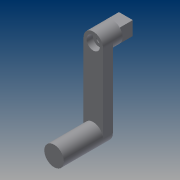
# Autodesk Inventor part: Crank
Saved by Autodesk Inventor 2016 (Build 200138000, 138)
## iProperties
Created: 2015-04-28
Part Number: Crank
Material: ABS Plastic
Document SubType Name: Modeling
Designer: Trevor
Density: 1.06 g/cm^3
Appearance: Smooth - White
d_key: 0.250 in
l_key: 0.265 in
t: 0.188 in
Author: Trevor
Autodesk Inventor part; units mm, degrees
ref_plane "YZ Plane" through (0, 0, 0) normal (1, 0, 0) x (0, 1, 0)
ref_plane "XZ Plane" through (0, 0, 0) normal (0, 1, 0) x (-1, 0, 0)
ref_plane "XY Plane" through (0, 0, 0) normal (0, 0, 1) x (1, 0, 0)
sketch "Sketch1" plane through (0, 0, 0) normal (0, 0, 1) x (1, 0, 0)
  line L0 (-3.3676, 3.3676) -> (3.3676, 3.3676)
  line L1 (3.3676, 3.3676) -> (3.3676, -3.3676)
  line L2 (3.3676, -3.3676) -> (-3.3676, -3.3676)
  line L3 (-3.3676, -3.3676) -> (-3.3676, 3.3676)
  line L4 (-3.3676, 3.3676) -> (3.3676, -3.3676) construction
  line L5 (3.3676, 3.3676) -> (-3.3676, -3.3676) construction
  point P0 (0, 0)
  dimension "d0" = 6.7352
  constraints: 12 end point, 2 midpoint, 2 parallel, 2 perpendicular, 1 horizontal
  measures "d0" distance of L0.end L1.end
extrude "Extrusion1" add sketch "Sketch1" along normal blind 6.35
sketch "Sketch2" plane through (0, 0, 6.35) normal (0, 0, 1) x (1, 0, 0)
  line L0 (3.3676, -3.3676) -> (3.3676, 3.3676) projected
  line L1 (-3.3676, -3.3676) -> (3.3676, -3.3676) projected
  line L2 (3.3676, 3.3676) -> (-3.3676, 3.3676) projected
  line L3 (-3.3676, 3.3676) -> (-3.3676, -3.3676) projected
  circle A0 centre (0, 0) radius 4.7625
  constraints: 1 coincident, 3 other
extrude "Extrusion2" add sketch "Sketch2" along normal blind 4.7625
sketch "Sketch3" plane through (0, 0, 11.1125) normal (0, 0, 1) x (1, 0, 0)
  circle A0 centre (0, 0) radius 4.7625 projected
  line L0 (0, 0) -> (0, -38.1) construction
  line L1 (-4.7625, 0) -> (-4.7625, -38.1)
  line L2 (4.7625, -38.1) -> (4.7625, 0)
  arc A1 (4.7625, 0) -> (-4.7625, 0) centre (0, 0) ccw
  arc A2 (-4.7625, -38.1) -> (4.7625, -38.1) centre (0, -38.1) ccw
  circle A3 centre (0, 0) radius 4.7625 projected
  point P0 (0, -19.05)
  dimension "d5" = 38.1
  constraints: 8 end point, 4 point on circle, 4 tangent, 2 centre point, 1 horizontal alignment, 1 midpoint, 1 parallel, 1 vertical, 1 other
  measures "d5" distance of L0.start L0.end
extrude "Extrusion3" add sketch "Sketch3" along normal blind 4.7625
sketch "Sketch4" plane through (0, 0, 15.875) normal (0, 0, 1) x (1, 0, 0)
  circle A0 centre (0, -38.1) radius 4.7625
  line L0 (4.7625, 0) -> (4.7625, -38.1) projected
  arc A1 (-4.7625, -38.1) -> (4.7625, -38.1) centre (0, -38.1) ccw projected
  line L1 (-4.7625, -38.1) -> (-4.7625, 0) projected
  arc A2 (4.7625, 0) -> (-4.7625, 0) centre (0, 0) ccw projected
  arc A3 (-4.7625, -38.1) -> (4.7625, -38.1) centre (0, -38.1) ccw projected
  constraints: 1 horizontal alignment, 3 other
extrude "Extrusion4" add sketch "Sketch4" along normal blind 19.05 contours A0
sketch "Sketch5" plane through (-3.3676, -3.3676, 0) normal (-1, 0, 0) x (0, 0, 1)
  point P0 (0, 3.3676)
sketch "Sketch6" plane through (0, 0, 15.875) normal (0, 0, 1) x (1, 0, 0)
  circle A0 centre (0, 0) radius 4.7625
  line L0 (4.7625, 0) -> (4.7625, -38.1) projected
  arc A1 (-4.7625, -38.1) -> (4.7625, -38.1) centre (0, -38.1) ccw projected
  arc A2 (4.7625, -38.1) -> (-4.7625, -38.1) centre (0, -38.1) ccw projected
  arc A3 (4.7625, 0) -> (-4.7625, 0) centre (0, 0) ccw projected
  line L1 (-4.7625, -38.1) -> (-4.7625, 0) projected
  constraints: 2 coincident, 1 horizontal alignment, 2 other
hole "Hole1" at (0, 0, 15.875) direction (0, 0, -1) diameter 3.4036 end through all counterbore diameter 6.5024 counterbore depth 2.9972 clearance for "Socket Head Cap Screw" size "M3" standard "Ansi Metric M Profile"
equation "\"d0\" = l_key"
equation "\"d1\" = d_key"
equation "\"d6\" = t"
equation "\"d8\" = 4 * t"
equation "\"l_key\" = 6.735192"
equation "\"d_key\" = 6.35"
equation "\"t\" = 4.7625"
body "Solid1"
